Autodesk Inventor part; units mm, degrees
(part 3 of 3)
  circle A133 centre (90.3659, -45.1111) radius 1.6
  circle A134 centre (45.1111, -90.3659) radius 1.6
  circle A135 centre (90.3659, 45.1111) radius 1.6
  circle A136 centre (45.1111, 90.3659) radius 1.6
  line L99 (41.3657, 27.2236) -> (27.2236, 41.3657) construction
  line L100 (34.2947, 34.2947) -> (55.1543, 55.1543) construction
  line L101 (46.669, 63.6396) -> (63.6396, 46.669) construction
  line L102 (0, 0) -> (0, -61.2072) construction
  circle A137 centre (0, -54) radius 1.6
  arc A138 (3.4868, -52.0398) -> (-3.4868, -52.0398) centre (0, -54) ccw
  line L103 (-0.6161, -51.9466) -> (-14.5119, -56.4463) construction
  line L104 (-5.1776, -53.4237) -> (-14.5119, -56.4463) construction
  line L105 (14.5119, -56.4463) -> (0.6161, -51.9466) construction
  line L106 (5.1776, -53.4237) -> (14.5119, -56.4463) construction
  arc A139 (0, -58) -> (3.8733, -53.0013) centre (0, -54) ccw construction
  arc A140 (-3.8733, -53.0013) -> (0, -58) centre (0, -54) ccw construction
  arc A141 (-5.1776, -53.4237) -> (-3.4868, -52.0398) centre (-6.1018, -50.5696) ccw
  arc A142 (3.4868, -52.0398) -> (5.1776, -53.4237) centre (6.1018, -50.5696) ccw
  line L107 (5.1776, -53.4237) -> (3.794, -57.2809)
  line L108 (3.794, -57.2809) -> (-2.6441, -58)
  line L109 (-2.6441, -58) -> (-5.1776, -53.4237)
  dimension "d114" = 3.2
  dimension "d117" = 64
  dimension "d118" = 3.2
  dimension "d119" = 54
  dimension "d120" = 8
  dimension "d121" = 3
  constraints: 20 end point, 15 centre point, 14 point on circle, 7 symmetric about line, 6 point on line, 4 midpoint, 4 tangent, 2 coincident, 2 collinear, 2 vertical, 1 equal radius, 1 horizontal, 7 other
  measures "d114" diameter of A129
  measures "d117" distance of A135.centre A136.centre
  measures "d118" diameter of A137
  measures "d119" distance of A137.centre point (0, 0)
  measures "d120" diameter of A138
  measures "d121" radius of A141
extrude "Выдавливание9" cut sketch "Эскиз6" against normal blind 10 contours A129 | A130 | A131 | A132 | A133 | A134 | A135 | A136 | A137
extrude "Выдавливание10" add sketch "Эскиз6" against normal blind 2 contours A142 L107 L108 L109 A141 A138
sketch "Эскиз7" plane through (0, 2, 0) normal (0, 1, 0) x (1, 0, 0)
  line L0 (-25, -33.1335) -> (25, -33.1335) construction
  line L1 (25, -33.1335) -> (25, -43.1335) construction
  line L2 (25, -43.1335) -> (-25, -43.1335) construction
  line L3 (-25, -43.1335) -> (-25, -33.1335) construction
  line L4 (0, 0) -> (0, -69.4501) construction
  circle A0 centre (21.9203, -43.1335) radius 1.6 construction
  circle A1 centre (-21.9203, -43.1335) radius 1.6 construction
  dimension "d124" = 50
  dimension "d125" = 10
  constraints: 10 end point, 2 parallel, 1 horizontal, 1 perpendicular, 1 point on line, 1 vertical, 1 other
  measures "d124" distance of L1.end L2.end
  measures "d125" distance of L0.end L1.end
